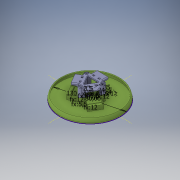
# Autodesk Inventor part: Stewart-Platform-Base-KST-DS215MG
Saved by Autodesk Inventor 2018.2 (Build 222227000, 227)
## iProperties
Created: 2018-02-17
Part Number: Stewart-Platform-Base-KST-DS215MG
Material: Generisch
Document SubType Name: Modeling
Designer: JochenAlt
Density: 1 g/cm^3
Appearance: Olivgrün
Author: JochenAlt
Autodesk Inventor part; units mm, degrees
ref_plane "YZ Plane" through (0, 0, 0) normal (1, 0, 0) x (0, 1, 0)
ref_plane "XZ Plane" through (0, 0, 0) normal (0, 1, 0) x (-1, 0, 0)
sketch "Skizze1" plane through (0, 0, 0) normal (0, 0, 1) x (1, 0, 0)
  line L0 (0, 91) -> (0, -91) construction
  line L1 (-91, 0) -> (91, 0) construction
  line L2 (-12, 26.62777) -> (-12, 33.52777)
  line L3 (12, 33.52777) -> (12, 26.62777)
  line L4 (29.060967, -2.921768) -> (35.035037, -6.371814)
  line L5 (23.032089, -27.15602) -> (17.058018, -23.705974)
  line L6 (-29.058682, -2.92183) -> (-35.035926, -6.373061)
  line L7 (-23.034664, -27.158241) -> (-17.057421, -23.707009)
  line L8 (12, 28.12777) -> (-12, 28.12777)
  line L9 (18.357601, -24.456488) -> (30.36055, -3.672282)
  line L10 (-12, 26.62777) -> (12, 26.62777)
  line L11 (-30.359169, -3.672724) -> (-18.357908, -24.457904)
  line L12 (22.531145, -28.023449) -> (35.534109, -5.507625)
  line L13 (-13.000757, 7.50546) -> (-13.000757, 33.52777)
  line L14 (13, 7.505898) -> (13, 33.52777)
  line L15 (-13.000757, 33.52777) -> (13, 33.52777)
  line L16 (13, 7.505898) -> (35.534109, -5.507625)
  line L17 (-13.000757, 7.50546) -> (-35.536301, -5.506453)
  line L18 (0, -15.011637) -> (-22.535165, -28.023332)
  line L19 (0, -15.011637) -> (22.531145, -28.023449)
  line L20 (-29.058682, -2.92183) -> (-17.057421, -23.707009)
  line L21 (17.058018, -23.705974) -> (29.060967, -2.921768)
  line L22 (-35.536301, -5.506453) -> (-22.535165, -28.023332)
  line L23 (-12, 6.92777) -> (-12, 26.62777)
  line L24 (12, 6.92777) -> (12, 26.62777)
  line L25 (12, 6.92777) -> (29.060967, -2.921768)
  line L26 (0, -13.858138) -> (17.058018, -23.705974)
  line L27 (0, -13.858138) -> (-17.057421, -23.707009)
  line L28 (-12, 6.92777) -> (-29.058682, -2.92183)
  circle A0 centre (0, 0) radius 28.12777 construction
  line L29 (-17.500547, 10.103314) -> (17.499453, 10.103314) construction
  circle A1 centre (-17.500547, 10.103314) radius 1.4
  circle A2 centre (17.499453, 10.103314) radius 1.4
  circle A3 centre (-17.500547, 10.103314) radius 2.15 construction
  circle A4 centre (17.499453, 10.103314) radius 2.15 construction
  line L30 (-15.350547, 8.862011) -> (-17.500547, 7.620708)
  line L31 (-17.500547, 7.620708) -> (-19.650547, 8.862011)
  line L32 (-19.650547, 8.862011) -> (-19.650547, 11.344617)
  line L33 (-19.650547, 11.344617) -> (-17.500547, 12.58592)
  line L34 (-17.500547, 12.58592) -> (-15.350547, 11.344617)
  line L35 (-15.350547, 11.344617) -> (-15.350547, 8.862011)
  line L36 (15.349453, 11.344617) -> (17.499453, 12.58592)
  line L37 (17.499453, 12.58592) -> (19.649453, 11.344617)
  line L38 (19.649453, 11.344617) -> (19.649453, 8.862011)
  line L39 (19.649453, 8.862011) -> (17.499453, 7.620708)
  line L40 (17.499453, 7.620708) -> (15.349453, 8.862011)
  line L41 (15.349453, 8.862011) -> (15.349453, 11.344617)
  arc A5 (-17.500547, 14.753314) -> (-21.527487, 7.778179) centre (-17.500547, 10.103314) ccw
  arc A6 (21.526204, 7.777852) -> (17.499453, 14.753314) centre (17.499453, 10.103314) ccw
  arc A7 (-4.028107, -22.529281) -> (4.023545, -22.529608) centre (-0.002187, -20.204735) ccw
  circle A8 centre (-0.002187, -20.204735) radius 2.15 construction
  line L42 (1.239116, -22.354735) -> (-1.24349, -22.354735)
  line L43 (-1.24349, -22.354735) -> (-2.484793, -20.204735)
  line L44 (-2.484793, -20.204735) -> (-1.24349, -18.054735)
  line L45 (-1.24349, -18.054735) -> (1.239116, -18.054735)
  line L46 (1.239116, -18.054735) -> (2.480419, -20.204735)
  line L47 (2.480419, -20.204735) -> (1.239116, -22.354735)
  line L48 (-17.500547, 10.103314) -> (-0.002187, -20.204735) construction
  line L49 (-0.002187, -20.204735) -> (17.499453, 10.103314) construction
  line L50 (-17.500547, 14.753314) -> (-13.000757, 14.753314)
  line L51 (-21.527487, 7.778179) -> (-19.277461, 3.881322)
  line L52 (13, 14.753314) -> (17.499453, 14.753314)
  line L53 (19.276031, 3.881469) -> (21.526204, 7.777852)
  line L54 (-4.028107, -22.529281) -> (-6.276325, -18.635557)
  line L55 (4.023545, -22.529608) -> (6.273067, -18.634354)
  circle A9 centre (-0.002187, -20.204735) radius 1.4
  line L56 (-17.057421, -23.707009) -> (-16.557921, -24.5721)
  line L57 (-29.058682, -2.92183) -> (-29.559057, -2.055221)
  line L58 (12, 26.62777) -> (13, 26.62777)
  line L59 (-12, 26.62777) -> (-13.000757, 26.62777)
  line L60 (29.060967, -2.921768) -> (29.560039, -2.05758)
  line L61 (17.058018, -23.705974) -> (16.557075, -24.573404)
  line L62 (0, -13.858138) -> (12, 6.92777)
  line L63 (12, 6.92777) -> (-12, 6.92777)
  line L64 (0, -13.858138) -> (-12, 6.92777)
  line L65 (6.273067, -18.634354) -> (6.773045, -17.768313)
  line L66 (19.276031, 3.881469) -> (18.776239, 3.015751)
  line L67 (13, 14.753314) -> (12, 14.753314)
  line L68 (-13.000757, 14.753314) -> (-12, 14.753314)
  line L69 (-19.277461, 3.881322) -> (-18.777086, 3.014714)
  line L70 (-6.276325, -18.635557) -> (-6.775824, -17.770466)
  circle A10 centre (-17.500547, 10.103314) radius 3.15
  circle A11 centre (17.499453, 10.103314) radius 3.15
  circle A12 centre (-0.002187, -20.204735) radius 3.15
  line L71 (-8, 12.42777) -> (-4, 12.42777)
  line L72 (-4, 12.42777) -> (-4, 15.42777)
  line L73 (-4, 15.42777) -> (-8, 15.42777)
  line L74 (-8, 15.42777) -> (-8, 12.42777)
  line L75 (4, 12.42777) -> (8, 12.42777)
  line L76 (8, 12.42777) -> (8, 15.42777)
  line L77 (8, 15.42777) -> (4, 15.42777)
  line L78 (4, 15.42777) -> (4, 12.42777)
  line L79 (6.763964, -13.142392) -> (9.362081, -14.642322)
  line L80 (9.362081, -14.642322) -> (11.361987, -11.178166)
  line L81 (11.361987, -11.178166) -> (8.76387, -9.678237)
  line L82 (8.76387, -9.678237) -> (6.763964, -13.142392)
  line L83 (12.763683, -2.749925) -> (15.361799, -4.249855)
  line L84 (15.361799, -4.249855) -> (17.361706, -0.785699)
  line L85 (17.361706, -0.785699) -> (14.763589, 0.71423)
  line L86 (14.763589, 0.71423) -> (12.763683, -2.749925)
  line L87 (-17.500547, 10.103314) -> (8.748633, -5.05071) construction
  line L88 (-11.361403, -11.178311) -> (-8.763368, -9.678241)
  line L89 (-8.763368, -9.678241) -> (-6.763193, -13.142429)
  line L90 (-6.763193, -13.142429) -> (-9.36131, -14.642359)
  line L91 (-9.36131, -14.642359) -> (-11.361403, -11.178311)
  line L92 (-15.361591, -4.250216) -> (-12.763474, -2.750287)
  line L93 (-12.763474, -2.750287) -> (-14.76338, 0.713869)
  line L94 (-14.76338, 0.713869) -> (-17.361497, -0.786061)
  line L95 (-17.361497, -0.786061) -> (-15.361591, -4.250216)
  line L96 (17.499453, 10.103314) -> (-8.750547, -5.05213) construction
  circle A13 centre (0, 0) radius 65
  point P0 (-15.350547, 10.103314)
  point P1 (15.349453, 10.103314)
  point P2 (1.859768, -21.279735)
  dimension "d217" = 4.3
  dimension "d212" = 24
  dimension "d213" = 5.4
  dimension "d214" = 1.5
  dimension "d215" = 1
  dimension "d216" = 2.8
  dimension "d218" = 2.5
  dimension "d219" = 35
  dimension "d220" = 26.6
  dimension "d221" = 1.5
  dimension "d222" = 5.5
  dimension "d223" = 4
  dimension "d224" = 12
  dimension "d225" = 3
  dimension "d228" = 5.5
  dimension "d229" = 12
  dimension "d230" = 30
  dimension "d231" = 30.0047
  dimension "d233" = 12
  dimension "d234" = 5.5
  dimension "d235" = 130
  constraints: 190 end point, 43 point on line, 29 perpendicular, 18 parallel, 16 coincident, 14 equal length, 11 centre point, 11 collinear, 9 horizontal, 9 tangent, 7 midpoint, 6 point on circle, 4 equal radius, 4 vertical, 2 horizontal alignment, 52 other
  measures "d212" distance between parallel lines of L3 L2
  measures "d213" distance between parallel lines of L8 L15
  measures "d214" distance between parallel lines of L10 L8
  measures "d215" distance between parallel lines of L14 L3
  measures "d216" diameter of A1
  measures "d219" distance of L29.start L29.end
  measures "d220" distance between parallel lines of L63 L15
  measures "d221" radial gap between concentric circles of A10 A5
  measures "d222" distance between parallel lines of L71 L63
  measures "d223" distance between parallel lines of L72 L74
  measures "d224" distance between parallel lines of L76 L72
  measures "d225" distance between parallel lines of L73 L71
  measures "d228" distance between parallel lines of L62 L82
  measures "d229" distance between parallel lines of L83 L79
  measures "d230" angle of L0 L48
  measures "d231" angle of L0 L49
  measures "d233" distance between parallel lines of L90 L92
  measures "d234" distance between parallel lines of L64 L93
  measures "d235" diameter of A13
extrude "Extrusion12" add sketch "Skizze1" along normal blind 2 contours L59 L13 L15 L2 | L10 L24 L63 L23 | L23 L68 L13 L59 | L2 L15 L3 L8 | L58 L14 L67 L24 | L3 L15 L14 L58 | L23 L28 L69 L17 L13 L68 | L67 L14 L16 L66 L25 L24 | L64 L27 L20 L28 | L13 L17 L51 A5 L50 | L25 L21 L26 L62 | L52 A6 L53 L16 L14 | L28 L57 L17 L69 | L26 L65 L19 L18 L70 L27 | L66 L16 L60 L25 | L6 L22 L17 L57 | L26 L61 L19 L65 | L70 L18 L56 L27 | L60 L16 L12 L4 | L11 L7 L22 L6 | L56 L18 L22 L7 | L5 L12 L19 L61 | L55 A7 L54 L18 L19 | L4 L12 L5 L9 | L30 L31 L32 L33 L34 L35 | L36 L37 L38 L39 L40 L41 | L42 L43 L44 L45 L46 L47 | A10 | A11 | A12 | L74 L73 L72 L71 | L78 L77 L76 L75 | L82 L81 L80 L79 | L86 L85 L84 L83 | L88 L89 L90 L91 | L95 L94 L93 L92 | A13
extrude "Extrusion5" add sketch "Skizze1" along normal blind 12 contours L59 L13 L15 L2 | L10 L24 L63 L23 | L23 L68 L13 L59 | L2 L15 L3 L8 | L58 L14 L67 L24 | L3 L15 L14 L58 | L23 L28 L69 L17 L13 L68 | L67 L14 L16 L66 L25 L24 | L64 L27 L20 L28 | L13 L17 L51 A5 L50 | L25 L21 L26 L62 | L52 A6 L53 L16 L14 | L28 L57 L17 L69 | L26 L65 L19 L18 L70 L27 | L66 L16 L60 L25 | L6 L22 L17 L57 | L26 L61 L19 L65 | L70 L18 L56 L27 | L60 L16 L12 L4 | L11 L7 L22 L6 | L56 L18 L22 L7 | L5 L12 L19 L61 | L55 A7 L54 L18 L19 | L4 L12 L5 L9 | L30 L31 L32 L33 L34 L35 | L36 L37 L38 L39 L40 L41 | L42 L43 L44 L45 L46 L47 | A10 | A11 | A12 | L74 L73 L72 L71 | L78 L77 L76 L75 | L82 L81 L80 L79 | L86 L85 L84 L83 | L88 L89 L90 L91 | L95 L94 L93 L92
extrude "Extrusion4" add sketch "Skizze1" along normal blind 16 contours L23 L28 L69 L17 L13 L68 | L67 L14 L16 L66 L25 L24 | L13 L17 L51 A5 L50 | L52 A6 L53 L16 L14 | L26 L65 L19 L18 L70 L27 | L55 A7 L54 L18 L19 | L30 L31 L32 L33 L34 L35 | L36 L37 L38 L39 L40 L41 | L42 L43 L44 L45 L46 L47 | A10 | A11 | A12
extrude "Extrusion13" cut sketch "Skizze1" against normal blind 1 from surface at 12 contours L10 L24 L63 L23 | L2 L15 L3 L8 | L64 L27 L20 L28 | L25 L21 L26 L62 | L20 L7 L11 L6 | L4 L9 L5 L21 | L11 L7 L22 L6 | L4 L12 L5 L9 | L74 L73 L72 L71 | L78 L77 L76 L75 | L82 L81 L80 L79 | L86 L85 L84 L83 | L88 L89 L90 L91 | L95 L94 L93 L92 | A13
extrude "Extrusion14" cut sketch "Skizze1" against normal blind 6 from surface at 16 contours L30 L31 L32 L33 L34 L35 | L36 L37 L38 L39 L40 L41 | L42 L43 L44 L45 L46 L47
fillet "Rundung4" radius 1 3 edges at (-12, 6.9278, 5.5) (12, 6.9278, 5.5) (0, -13.8581, 5.5)
fillet "Rundung4" radius 0.75 12 edges at (20.5305, 2.003, 11) (12, 16.7778, 11) (-20.5293, 2.003, 11) (-12, 16.7778, 11) (-8.5287, -18.7826, 11) (8.529, -18.7821, 11) (-32.6975, -5.0229, 11) (-20.6963, -25.8081, 11) (32.6978, -5.022, 11) (20.6948, -25.8063, 11) (12, 30.8278, 11) (-12, 30.8278, 11)
sketch "Skizze10" plane through (0, 0, 0) normal (0, 1, 0) x (-1, 0, 0)
  line L0 (-84.113255, 0) -> (84.679529, 0) construction
  line L1 (0, -2.169181) -> (0, 13.015086) construction
  line L2 (65, 0) -> (65, 2)
  arc A0 (65, 2) -> (62.688578, 10) centre (50, 2) ccw
  line L3 (65, 2) -> (65, 0)
  line L4 (-65, 0) -> (65, 0)
  line L5 (63, 0) -> (63, 2)
  line L6 (65, 2) -> (-65, 2) construction
  line L7 (65, 0) -> (65, 2) construction
  line L8 (91, 0) -> (-91, 0) construction
  arc A1 (63, 2) -> (60.996767, 8.933333) centre (50, 2) ccw
  arc A2 (62.688578, 10) -> (60.996767, 8.933333) centre (61.842672, 9.466667) ccw
  line L9 (0, -2.169181) -> (0, 13.015086)
  point P0 (0, 0)
  dimension "d245" = 1
  dimension "d246" = 15
  dimension "d247" = 10
  constraints: 6 point on circle, 4 end point, 3 centre point, 3 point on line, 3 tangent, 1 collinear, 1 concentric, 1 perpendicular, 1 other
  measures "d245" radius of A2
  measures "d246" radius of A0
  measures "d247" distance from line of L0 A0.end
revolve "Umdrehung2" add sketch "Skizze10" angle 360 about axis through (0, 0, -10) along (0, 0, 1)
ref_plane "Arbeitsebene4" through (0, 0, 35) normal (0, 0, 1) x (1, 0, 0)
extrude "Extrusion15" add sketch "Skizze1" against normal blind 2 from surface at 35 separate body contours L10 L24 L63 L23 | L23 L68 L13 L59 | L58 L14 L67 L24 | L23 L28 L69 L17 L13 L68 | L67 L14 L16 L66 L25 L24 | L64 L27 L20 L28 | L13 L17 L51 A5 L50 | L25 L21 L26 L62 | L52 A6 L53 L16 L14 | L28 L57 L17 L69 | L26 L65 L19 L18 L70 L27 | L66 L16 L60 L25 | L26 L61 L19 L65 | L70 L18 L56 L27 | L55 A7 L54 L18 L19 | L30 L31 L32 L33 L34 L35 | L36 L37 L38 L39 L40 L41 | L42 L43 L44 L45 L46 L47 | A10 | A11 | A12
extrude "Extrusion16" add sketch "Skizze1" against normal blind 2 from surface at 33 contours L23 L68 L13 L59 | L58 L14 L67 L24 | L23 L28 L69 L17 L13 L68 | L67 L14 L16 L66 L25 L24 | L13 L17 L51 A5 L50 | L52 A6 L53 L16 L14 | L28 L57 L17 L69 | L26 L65 L19 L18 L70 L27 | L66 L16 L60 L25 | L26 L61 L19 L65 | L70 L18 L56 L27 | L55 A7 L54 L18 L19 | L30 L31 L32 L33 L34 L35 | L36 L37 L38 L39 L40 L41 | L42 L43 L44 L45 L46 L47 | A10 | A11 | A12 bodies 2
extrude "Extrusion17" add sketch "Skizze1" against normal up to surface (15 mm away) from surface at 31 contours L23 L28 L69 L17 L13 L68 | L67 L14 L16 L66 L25 L24 | L13 L17 L51 A5 L50 | L52 A6 L53 L16 L14 | L26 L65 L19 L18 L70 L27 | L55 A7 L54 L18 L19 | L30 L31 L32 L33 L34 L35 | L36 L37 L38 L39 L40 L41 | L42 L43 L44 L45 L46 L47 | A10 | A11 | A12 bodies 2
fillet "Rundung6" radius 1 3 edges at (12, 6.9278, 34) (-12, 6.9278, 34) (0, -13.8581, 34)
fillet "Rundung6" radius 0.75 6 edges at (8.529, -18.7821, 33) (-8.5287, -18.7826, 33) (-12, 16.7778, 33) (12, 16.7778, 33) (20.5305, 2.003, 33) (-20.5293, 2.003, 33)
fillet "Rundung6" radius 2 6 edges at (-11.4171, -21.6038, 35) (11.4151, -21.6039, 35) (24.418, 0.9119, 35) (13, 20.6905, 35) (-13.0008, 20.6905, 35) (-24.4183, 0.9131, 35)
fillet "Rundung6" radius 1 12 edges at (20.4011, 5.8297, 35) (15.2497, 14.7533, 35) (21.5266, 12.4281, 35) (-21.5276, 12.4282, 35) (-20.4025, 5.8298, 35) (-15.2507, 14.7533, 35) (-0.0024, -24.8536, 35) (-5.1522, -20.5824, 35) (5.1483, -20.582, 35) (6, -3.4652, 35) (-6, -3.4652, 35) (0, 6.9278, 35)
fillet "Rundung6" radius 1 9 edges at (0, -13.6045, 11.2197) (0, -13.8581, 13.875) (11.7803, 6.8009, 11.2197) (12, 6.9278, 13.875) (-11.7803, 6.8009, 11.2197) (-12, 6.9278, 13.875) (0, -13.8581, 24.5) (12, 6.9278, 24.5) (-12, 6.9278, 24.5)
fillet "Rundung6" radius 5 12 edges at (12.5, 14.7533, 12) (-12.5004, 14.7533, 12) (-19.0273, 3.448, 12) (-6.5261, -18.203, 12) (6.5231, -18.2013, 12) (19.0261, 3.4486, 12) (12.5, 14.7533, 31) (-12.5004, 14.7533, 31) (19.0261, 3.4486, 31) (6.5231, -18.2013, 31) (-6.5261, -18.203, 31) (-19.0273, 3.448, 31)
extrude "Extrusion18" cut sketch "Skizze1" against normal blind 2 from surface at 35 contours L30 L31 L32 L33 L34 L35 | L36 L37 L38 L39 L40 L41 | L42 L43 L44 L45 L46 L47 | A10 | A11 | A12 bodies 2
equation "\"d44\" = d21"
equation "\"d21\" = 0.3"
